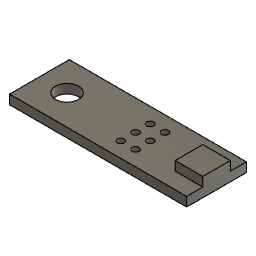
Fast Light Board With 90 Degree Header (Autodesk Fusion 360 archive; units mm, degrees)
design "Fast Light Board"
part number: fast-rgb-led-insert
Autodesk Fusion 360 part; units mm, degrees
sketch "Sketch1" plane through (0, 0, 0) normal (0, 1, 0) x (1, 0, 0) in component "Fast Light Board"
  line L0 (0, 0) -> (30.5594, 0)
  line L1 (30.5594, 0) -> (30.5594, 10.3188)
  line L2 (30.5594, 10.3188) -> (0, 10.3188)
  line L3 (0, 10.3188) -> (0, 0)
  circle A0 centre (4.7625, 5.1594) radius 1.9844
  dimension "d1" = 10.3188
  dimension "d2" = 30.5594
  dimension "d4" = 3.9688
  constraint horizontal L0
  constraint vertical L1
  constraint horizontal L2
  constraint vertical L3
  constraint coincident L0.start L3.end
  measures "d1" distance of L0.start L2.end
  measures "d2" distance of L0.start L0.end
  measures "d4" diameter of A0
extrude "Extrude1" add sketch "Sketch1" along normal blind 1.5875 in component "Fast Light Board"
sketch "Sketch2" plane through (0, 1.5875, 0) normal (0, 1, 0) x (-1, 0, 0) in component "Fast Light Board"
  circle A0 centre (-4.7625, -5.1594) radius 1.9844
  line L0 (0, -10.3188) -> (0, 0)
  line L1 (0, 0) -> (-30.5594, 0)
  line L2 (-30.5594, 0) -> (-30.5594, -10.3188)
  line L3 (-30.5594, -10.3188) -> (0, -10.3188)
  line L4 (-25.7969, -5.1594) -> (-25.7969, -7.5406)
  line L5 (-25.7969, -7.5406) -> (-30.5594, -7.5406)
  line L6 (-30.5594, -5.1594) -> (-30.5594, -7.5406)
  line L7 (-30.5594, -5.1594) -> (-30.5594, -2.7781)
  line L8 (-30.5594, -2.7781) -> (-25.7969, -2.7781)
  line L9 (-25.7969, -2.7781) -> (-25.7969, -5.1594)
  dimension "d7" = 4.7625
  constraint midpoint L2 L6.start
  constraint coincident L2 L5.end
  constraint perpendicular L2 L5
  constraint perpendicular L4 L8
  measures "d7" distance of L6.start L4.start
extrude "Extrude2" add sketch "Sketch2" along normal blind 1.5875 contours L2 L4 L5 L6 L7 L8 L9 in component "Fast Light Board"
sketch "Sketch3" plane through (0, 1.5875, 0) normal (0, 1, 0) x (-1, 0, 0) in component "Fast Light Board"
  line L0 (-25.7969, -7.5406) -> (-30.5594, -7.5406)
  line L1 (-30.5594, -7.5406) -> (-30.5594, -10.3188)
  line L2 (-30.5594, -10.3188) -> (0, -10.3188)
  line L3 (0, -10.3188) -> (0, 0)
  line L4 (0, 0) -> (-30.5594, 0)
  line L5 (-30.5594, 0) -> (-30.5594, -2.7781)
  line L6 (-30.5594, -2.7781) -> (-25.7969, -2.7781)
  line L7 (-25.7969, -2.7781) -> (-25.7969, -7.5406)
  circle A0 centre (-4.7625, -5.1594) radius 1.9844
  line L8 (-30.5594, -5.1594) -> (-17.8594, -5.1594)
  line L9 (-17.8594, -5.1594) -> (-19.1294, -5.1594)
  circle A1 centre (-19.1294, -5.1594) radius 0.5953
  circle A2 centre (-16.5894, -5.1594) radius 0.5953
  circle A3 centre (-19.1294, -7.6994) radius 0.5953
  circle A4 centre (-16.5894, -7.6994) radius 0.5953
  circle A5 centre (-16.5894, -2.6194) radius 0.5953
  circle A6 centre (-19.1294, -2.6194) radius 0.5953
  dimension "d12" = 12.7
  dimension "d13" = 1.27
  dimension "d14" = 1.1906
  dimension "d15" = 1.1906
  dimension "d16" = 1.1906
  dimension "d17" = 1.1906
  dimension "d18" = 1.1906
  dimension "d19" = 1.1906
  constraint perpendicular L7 L8
  constraint parallel L8 L9
  constraint coincident L9.end A1.centre
  measures "d12" distance of L8.start L8.end
  measures "d13" distance of L8.end L9.end
  measures "d14" diameter of A1
  measures "d15" diameter of A2
  measures "d16" diameter of A3
  measures "d17" diameter of A4
  measures "d18" diameter of A6
  measures "d19" diameter of A5
extrude "Extrude3" cut sketch "Sketch3" against normal blind 1.5875 contours L8 L9 A1 | L8 L9 A1 | A2 | A3 | A4 | A5 | A6 in component "Fast Light Board"
component "Fast Light Board" placed x (1, 0, 0) y (0, 1, 0) z (0, 0, 1) at (0, 0, 0)
equation "d1 = ( 13 / 32 ) * 1 in"
equation "d2 = 1 13/64\""
equation "d4 = ( 5 / 32 ) * 1 in"
equation "d5 = ( 1 / 16 ) * 1 in"
equation "d7 = ( 3 / 16 ) * 1 in"
equation "d10 = ( 1 / 16 ) * 1 in"
equation "d14 = ( 3 / 64 ) * 1 in"
equation "d15 = ( 3 / 64 ) * 1 in"
equation "d16 = ( 3 / 64 ) * 1 in"
equation "d17 = ( 3 / 64 ) * 1 in"
equation "d18 = ( 3 / 64 ) * 1 in"
equation "d19 = ( 3 / 64 ) * 1 in"
equation "d20 = ( -1 / 16 ) * 1 in"
